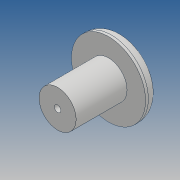
# Autodesk Inventor part: remache
Saved by Autodesk Inventor 2017 (Build 210142000, 142)
## iProperties
Created: 2017-08-05
Part Number: remache
Material: Generic
Document SubType Name: Modeling
Designer: leo
Density: 1 g/cm^3
Appearance: Default
Author: leo
Autodesk Inventor part; units mm, degrees
ref_plane "YZ Plane" through (0, 0, 0) normal (1, 0, 0) x (0, 1, 0)
ref_plane "XZ Plane" through (0, 0, 0) normal (0, 1, 0) x (-1, 0, 0)
ref_plane "XY Plane" through (0, 0, 0) normal (0, 0, 1) x (1, 0, 0)
sketch "Sketch1" plane through (0, 0, 0) normal (0, 0, 1) x (1, 0, 0)
  line L0 (0.35, 0) -> (0.35, 7)
  line L1 (0.35, 7) -> (2.8418, 7)
  arc A0 (4, 5.8) -> (2.8418, 7) centre (2.8418, 5.8411) ccw
  line L2 (4, 5.8) -> (4, 5.5)
  line L3 (4, 5.5) -> (2, 5.5)
  line L4 (2, 5.5) -> (2, 0)
  line L5 (2, 0) -> (0.35, 0)
  line L6 (0, 0) -> (0, 7) construction
  dimension "d0" = 4
  dimension "d1" = 0.7
  dimension "d2" = 7
  dimension "d3" = 1.5
  dimension "d4" = 8
  dimension "d5" = 0.3
  constraints: 14 end point, 6 perpendicular, 2 point on circle, 2 point on line, 1 centre point, 1 tangent, 1 vertical
  measures "d0" diameter of L4 L6
  measures "d1" diameter of L0 L6
  measures "d2" distance of L0.start L0.end
  measures "d3" distance between parallel lines of L1 L3
  measures "d4" diameter of L2 L6
  measures "d5" distance of L2.start L2.end
revolve "Revolution1" add sketch "Sketch1" angle 360 about axis through (0, 0, 0) along (0, 1, 0)
body "Solid1"
